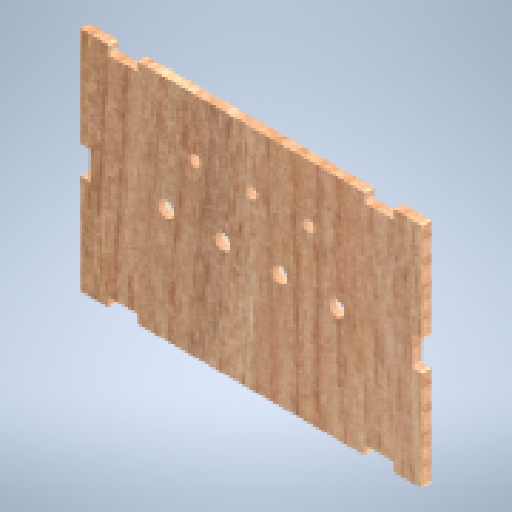
# Autodesk Inventor part: Front Panel
Saved by Autodesk Inventor 2023.1 (Build 271208000, 208)
## iProperties
Created: 2022-07-14
Part Number: Front Panel
Material: Wood (Birch)
Document SubType Name: Modeling
Designer: Eli
Density: 0.55 g/cm^3
Appearance: Birch - Natural Polished
Author: Eli
Autodesk Inventor part; units mm, degrees
ref_plane "YZ Plane" through (0, 0, 0) normal (1, 0, 0) x (0, 1, 0)
ref_plane "XZ Plane" through (0, 0, 0) normal (0, 1, 0) x (-1, 0, 0)
ref_plane "XY Plane" through (0, 0, 0) normal (0, 0, 1) x (1, 0, 0)
sketch "Sketch1" plane through (0, 0, 0) normal (0, 0, 1) x (1, 0, 0)
  line L0 (0, 0) -> (152.4, 0)
  line L1 (152.4, 0) -> (152.4, 101.6)
  line L2 (152.4, 101.6) -> (0, 101.6)
  line L3 (0, 101.6) -> (0, 0)
  circle A0 centre (38.1, 50.8) radius 3.5
  circle A1 centre (63.5, 50.8) radius 3.5
  circle A2 centre (88.9, 50.8) radius 3.5
  circle A3 centre (114.3, 50.8) radius 3.5
  circle A4 centre (50.8, 76.2) radius 2.5
  circle A5 centre (76.2, 76.2) radius 2.5
  circle A6 centre (101.6, 76.2) radius 2.5
  line L4 (12.7, 101.6) -> (25.4, 101.6)
  line L5 (25.4, 101.6) -> (25.4, 97.6)
  line L6 (25.4, 97.6) -> (12.7, 97.6)
  line L7 (12.7, 97.6) -> (12.7, 101.6)
  line L8 (139.7, 101.6) -> (127, 101.6)
  line L9 (127, 101.6) -> (127, 97.6)
  line L10 (127, 97.6) -> (139.7, 97.6)
  line L11 (139.7, 97.6) -> (139.7, 101.6)
  line L12 (139.7, 0) -> (127, 0)
  line L13 (127, 0) -> (127, 4)
  line L14 (127, 4) -> (139.7, 4)
  line L15 (139.7, 4) -> (139.7, 0)
  line L16 (12.7, 0) -> (25.4, 0)
  line L17 (25.4, 0) -> (25.4, 4)
  line L18 (25.4, 4) -> (12.7, 4)
  line L19 (12.7, 4) -> (12.7, 0)
  line L20 (0, 57.15) -> (4, 57.15)
  line L21 (4, 57.15) -> (4, 44.45)
  line L22 (4, 44.45) -> (0, 44.45)
  line L23 (0, 44.45) -> (0, 57.15)
  line L24 (152.4, 57.15) -> (148.4, 57.15)
  line L25 (148.4, 57.15) -> (148.4, 44.45)
  line L26 (148.4, 44.45) -> (152.4, 44.45)
  line L27 (152.4, 44.45) -> (152.4, 57.15)
  point P0 (76.2, 0)
  point P1 (76.2, 101.6)
  point P2 (12.7, 99.6)
  point P3 (139.7, 99.6)
  point P4 (12.7, 2)
  point P5 (0, 50.8)
  point P6 (4, 50.8)
  point P7 (148.4, 50.8)
  point P8 (152.4, 50.8)
  point P9 (0, 50.8)
  dimension "d0" = 152.4
  dimension "d1" = 101.6
  dimension "d2" = 7
  dimension "d5" = 25.4
  dimension "d10" = 12.7
  dimension "d11" = 50.8
  dimension "d12" = 5
  dimension "d15" = 25.4
  dimension "d20" = 25.4
  dimension "d21" = 12.7
  dimension "d22" = 4
  dimension "d23" = 12.7
  dimension "d24" = 12.7
  dimension "d25" = 4
  dimension "d26" = 12.7
  dimension "d27" = 4
  dimension "d28" = 12.7
  dimension "d29" = 4
  dimension "d30" = 4
  dimension "d31" = 12.7
  dimension "d32" = 4
  dimension "d33" = 12.7
  dimension "d34" = 12.7
  dimension "d35" = 12.7
  constraints: 56 end point, 14 parallel, 10 midpoint, 9 horizontal, 7 centre point, 7 perpendicular, 7 point on line, 3 horizontal alignment, 1 vertical alignment, 10 other
  measures "d0" distance of L2.end L1.end
  measures "d1" distance of L1.end L0.end
  measures "d2" diameter of A0
  measures "d5" distance of A0.centre A1.centre
  measures "d10" horizontal distance of point (76.2, 0) A1.centre
  measures "d11" distance from line of L0 A1.centre
  measures "d12" diameter of A4
  measures "d15" distance of A4.centre A5.centre
  measures "d20" vertical distance of A5.centre A1.centre
  measures "d21" distance of L5.end L6.end
  measures "d22" distance of L4.end L5.end
  measures "d23" distance from line of L3 point (12.7, 99.6)
  measures "d24" distance of L10.end L9.end
  measures "d25" distance of L9.end L8.end
  measures "d26" distance of L13.end L14.end
  measures "d27" distance of L12.end L13.end
  measures "d28" distance of L18.end L17.end
  measures "d29" distance of L17.end L16.end
  measures "d30" distance of L21.end L22.end
  measures "d31" distance of L20.end L21.end
  measures "d32" distance of L26.end L25.end
  measures "d33" distance of L25.end L24.end
  measures "d34" distance from line of L1 point (139.7, 99.6)
  measures "d35" distance from line of L3 point (12.7, 2)
extrude "Extrusion1" add sketch "Sketch1" along normal blind 4 contours L3 L22 L21 L20 L2 L7 L6 L5 L9 L10 L11 L1 L24 L25 L26 L0 L15 L14 L13 L17 L18 L19
body "Solid1"
